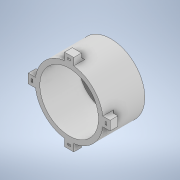
# Autodesk Inventor part: Weight_case
Saved by Autodesk Inventor 2020 (Build 240168000, 168)
## iProperties
Created: 2019-09-30
Part Number: Weight_case
Material: 일반
Document SubType Name: Modeling
Designer: Knowblesse
Density: 1 g/cm^3
Appearance: 기본값
Author: Knowblesse
## iProperties of the stored document _3D 인쇄.ipt
Created: 2019-09-30
Part Number: _3D 인쇄
Material: 일반
Document SubType Name: Modeling
Designer: Knowblesse
Density: 1 g/cm^3
Appearance: 기본값
Author: Knowblesse
Autodesk Inventor part; units mm, degrees
ref_plane "YZ Plane" through (0, 0, 0) normal (1, 0, 0) x (0, 1, 0)
ref_plane "XZ Plane" through (0, 0, 0) normal (0, 1, 0) x (-1, 0, 0)
ref_plane "XY Plane" through (0, 0, 0) normal (0, 0, 1) x (1, 0, 0)
sketch "스케치1" plane through (0, 0, 0) normal (0, 0, 1) x (1, 0, 0)
  circle A0 centre (0, 0) radius 22
  dimension "d0" = 44
  constraints: 1 centre point, 1 coincident
  measures "d0" diameter of A0
extrude "돌출1" add sketch "스케치1" along normal blind 2
sketch "스케치2" plane through (0, 0, 2) normal (0, 0, 1) x (1, 0, 0)
  circle A0 centre (0, 0) radius 22
  circle A1 centre (0, 0) radius 19
  circle A2 centre (0, 0) radius 22 projected
  dimension "d7" = 38
  constraints: 2 centre point, 2 coincident, 1 concentric
  measures "d7" diameter of A1
extrude "돌출2" add sketch "스케치2" along normal blind 25
sketch "스케치3" plane through (0, 0, 27) normal (0, 0, 1) x (1, 0, 0)
  line L0 (-3, -26.5) -> (3, -26.5)
  line L1 (3, -26.5) -> (3, -20.5)
  line L2 (3, -20.5) -> (-3, -20.5)
  line L3 (-3, -20.5) -> (-3, -26.5)
  circle A0 centre (0, 0) radius 19 construction
  line L4 (0, -19) -> (0, -22) construction
  circle A1 centre (0, 0) radius 22 construction
  line L5 (-1, -24.5) -> (1, -24.5)
  line L6 (1, -24.5) -> (1, -23.5)
  line L7 (1, -23.5) -> (-1, -23.5)
  line L8 (-1, -23.5) -> (-1, -24.5)
  point P0 (0, -20.5)
  point P1 (0, -23.5)
  dimension "d8" = 6
  dimension "d9" = 6
  dimension "d10" = 2
  dimension "d11" = 2
  dimension "d12" = 1
  constraints: 18 end point, 4 parallel, 4 vertical alignment, 3 midpoint, 2 horizontal, 2 perpendicular, 1 vertical, 2 other
  measures "d8" distance of L2.end L0.start
  measures "d9" distance of L0.start L0.end
  measures "d10" distance between parallel lines of L3 L8
  measures "d11" distance between parallel lines of L0 L5
  measures "d12" distance of L5.end L6.end
extrude "돌출3" add sketch "스케치3" against normal blind 5
chamfer "모따기1" distance 2 angle 45 1 edges at (0, -22, 22)
pattern_circular "원형 패턴1" count 4 over 360 about axis through (0, 0, 2) along (0, 0, 1) of "돌출3", "모따기1"
